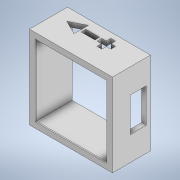
# Autodesk Inventor part: Case
Saved by Autodesk Inventor 2020.1 (Build 241239000, 239)
## iProperties
Created: 2019-09-02
Part Number: Case
Material: Generic
Document SubType Name: Modeling
Designer: matteo.spadetto-1
Density: 1 g/cm^3
Appearance: Default
Author: matteo.spadetto-1
Autodesk Inventor part; units mm, degrees
ref_plane "YZ Plane" through (0, 0, 0) normal (1, 0, 0) x (0, 1, 0)
ref_plane "XZ Plane" through (0, 0, 0) normal (0, 1, 0) x (-1, 0, 0)
ref_plane "XY Plane" through (0, 0, 0) normal (0, 0, 1) x (1, 0, 0)
sketch "Sketch2" plane through (0, 0, 0) normal (0, 0, 1) x (1, 0, 0)
  line L0 (0, 0) -> (73, 0)
  line L1 (73, 0) -> (73, 73)
  line L2 (73, 73) -> (0, 73)
  line L3 (0, 73) -> (0, 0)
  dimension "d2" = 73
  dimension "d3" = 73
  constraints: 8 end point, 2 parallel, 1 horizontal, 1 perpendicular
  measures "d2" distance of L2.end L1.end
  measures "d3" distance of L1.end L0.end
extrude "Extrusion1" add sketch "Sketch2" along normal blind 20
sketch "Sketch3" plane through (0, 0, 0) normal (0, 0, -1) x (-1, 0, 0)
  line L0 (-73, 73) -> (0, 73) projected
  line L1 (0, 73) -> (0, 0) projected
  line L2 (-73, 73) -> (0, 73)
  line L3 (0, 73) -> (0, 0)
  line L4 (0, 0) -> (-73, 0)
  line L5 (-73, 0) -> (-73, 73)
  line L6 (-69, 69) -> (-4, 69)
  line L7 (-4, 69) -> (-4, 4)
  line L8 (-4, 4) -> (-69, 4)
  line L9 (-69, 4) -> (-69, 69)
  dimension "d6" = 4
  constraints: 16 end point, 4 parallel, 2 perpendicular, 1 horizontal, 3 other
  measures "d6" distance between parallel lines of L5 L9
extrude "Extrusion2" cut sketch "Sketch3" against normal blind 20 contours L6 L7 L8 L9
sketch "Sketch4" plane through (0, 0, 20) normal (0, 0, 1) x (1, 0, 0)
  line L0 (4, 4) -> (4, 69) projected
  line L1 (69, 69) -> (69, 4) projected
  line L2 (4, 4) -> (69, 4)
  line L3 (69, 4) -> (69, 69)
  line L4 (69, 69) -> (4, 69)
  line L5 (4, 69) -> (4, 4)
  line L6 (5, 68) -> (68, 68)
  line L7 (68, 68) -> (68, 5)
  line L8 (68, 5) -> (5, 5)
  line L9 (5, 5) -> (5, 68)
  point P0 (0, 0)
  point P1 (69, 4)
  point P2 (4, 69)
  dimension "d9" = 1
  constraints: 16 end point, 4 parallel, 2 perpendicular, 1 horizontal, 3 other
  measures "d9" distance between parallel lines of L4 L6
extrude "Extrusion3" add sketch "Sketch4" against normal blind 1
sketch "Sketch5" plane through (0, 0, 0) normal (0, 0, -1) x (-1, 0, 0)
  line L0 (-4, 69) -> (-4, 4) projected
  line L1 (-4, 4) -> (-69, 4) projected
  line L2 (-4, 69) -> (-69, 69)
  line L3 (-69, 69) -> (-69, 4)
  line L4 (-69, 4) -> (-4, 4)
  line L5 (-4, 4) -> (-4, 69)
  line L6 (0, 73) -> (0, 0) projected
  line L7 (0, 0) -> (-73, 0) projected
  line L8 (0, 73) -> (-73, 73)
  line L9 (-73, 73) -> (-73, 0)
  line L10 (-73, 0) -> (0, 0)
  line L11 (0, 0) -> (0, 73)
  constraints: 16 end point, 4 parallel, 2 horizontal, 2 perpendicular
extrude "Extrusion4" add sketch "Sketch5" along normal blind 13.5
sketch "Sketch7" plane through (73, 0, 20) normal (1, 0, 0) x (0, 0, -1)
  line L0 (33.5, 69) -> (33.5, 4) projected
  line L1 (29.6, 36.5) -> (29.6, 51.5)
  line L2 (29.6, 51.5) -> (15.6, 51.5)
  line L3 (15.6, 51.5) -> (15.6, 21.5)
  line L4 (15.6, 21.5) -> (29.6, 21.5)
  line L5 (29.6, 21.5) -> (29.6, 36.5)
  point P0 (20, 0)
  dimension "d57" = 2.5
  dimension "d43" = 15
  dimension "d44" = 14
  dimension "d45" = 30
  constraints: 10 end point, 3 perpendicular, 1 point on line, 1 vertical
  measures "d43" distance of L1.start L1.end
  measures "d44" distance of L1.end L2.end
  measures "d45" distance of L2.end L3.end
extrude "Extrusion5" cut sketch "Sketch7" against normal blind 4
sketch "Sketch8" plane through (0, 0, 20) normal (-1, 0, 0) x (0, 0, 1)
  line L0 (-26.5, 65) -> (-24, 65)
  circle A0 centre (-24, 65) radius 1.5
  point P0 (-20, 0)
  point P1 (-33.5, 69)
  constraints: 2 end point, 1 centre point, 1 coincident, 1 horizontal
extrude "Extrusion6" cut sketch "Sketch8" against normal blind 4
sketch "Sketch9" plane through (0, 0, 20) normal (-1, 0, 0) x (0, 0, 1)
  line L0 (-33.5, 73) -> (0, 73) projected
  line L1 (-33.5, 73) -> (-33.5, 66.5)
  line L2 (-33.5, 66.5) -> (-31.5, 66.5)
  line L3 (-31.5, 66.5) -> (-31.5, 63.5)
  line L4 (-31.5, 63.5) -> (-33.5, 63.5)
  line L5 (-33.5, 63.5) -> (-33.5, 66.5)
  point P0 (-20, 0)
  dimension "d55" = 2
  dimension "d56" = 3
  constraints: 10 end point, 2 parallel, 1 horizontal, 1 perpendicular, 1 vertical
  measures "d55" distance of L3.end L4.end
  measures "d56" distance of L2.end L3.end
extrude "Extrusion7" cut sketch "Sketch9" against normal blind 2.5
sketch "Sketch10" plane through (0, 73, 20) normal (0, 1, 0) x (1, 0, 0)
  line L0 (0, 0) -> (73, 0) projected
  line L1 (73, 33.5) -> (0, 33.5) projected
  line L2 (0, 33.5) -> (0, 0) projected
  line L3 (4, 33.5) -> (4, 1) projected
  line L4 (51.2, 20.4) -> (47.2, 20.4)
  line L5 (47.2, 20.4) -> (47.2, 16.4)
  line L6 (47.2, 16.4) -> (42.8, 16.4)
  line L7 (42.8, 16.4) -> (42.8, 20.4)
  line L8 (42.8, 20.4) -> (38.8, 20.4)
  line L9 (38.8, 20.4) -> (38.8, 24.8)
  line L10 (38.8, 24.8) -> (42.8, 24.8)
  line L11 (42.8, 24.8) -> (42.8, 28.8)
  line L12 (42.8, 28.8) -> (47.2, 28.8)
  line L13 (47.2, 28.8) -> (47.2, 24.8)
  line L14 (47.2, 24.8) -> (51.2, 24.8)
  line L15 (51.2, 24.8) -> (51.2, 20.4)
  line L16 (24.8, 20.4) -> (37.2, 20.4)
  line L17 (37.2, 20.4) -> (37.2, 24.8)
  line L18 (37.2, 24.8) -> (24.8, 24.8)
  line L19 (24.8, 24.8) -> (24.8, 20.4)
  line L20 (10.161, 22.4041) -> (23.2, 28.9236)
  line L21 (23.2, 28.9236) -> (23.2, 15.8846)
  line L22 (23.2, 15.8846) -> (10.161, 22.4041)
  line L23 (23.1, 28.7618) -> (10.3846, 22.4041)
  line L24 (10.3846, 22.4041) -> (23.1, 16.0464)
  line L25 (23.1, 16.0464) -> (23.1, 28.7618)
  line L26 (24.9, 24.7) -> (37.1, 24.7)
  line L27 (37.1, 24.7) -> (37.1, 20.5)
  line L28 (37.1, 20.5) -> (24.9, 20.5)
  line L29 (24.9, 20.5) -> (24.9, 24.7)
  line L30 (42.9, 24.7) -> (38.9, 24.7)
  line L31 (38.9, 24.7) -> (38.9, 20.5)
  line L32 (38.9, 20.5) -> (42.9, 20.5)
  line L33 (42.9, 20.5) -> (42.9, 16.5)
  line L34 (42.9, 16.5) -> (47.1, 16.5)
  line L35 (47.1, 16.5) -> (47.1, 20.5)
  line L36 (47.1, 20.5) -> (51.1, 20.5)
  line L37 (51.1, 20.5) -> (51.1, 24.7)
  line L38 (51.1, 24.7) -> (47.1, 24.7)
  line L39 (47.1, 24.7) -> (47.1, 28.7)
  line L40 (47.1, 28.7) -> (42.9, 28.7)
  line L41 (42.9, 28.7) -> (42.9, 24.7)
  point P0 (0, 20)
  dimension "d95" = 0.1
  dimension "d96" = 0.1
  dimension "d97" = 0.1
  constraints: 76 end point, 8 perpendicular, 2 parallel, 16 other
  measures "d95" distance between parallel lines of L20 L23
  measures "d96" distance between parallel lines of L18 L26
  measures "d97" distance between parallel lines of L10 L30
extrude "Extrusion8" cut sketch "Sketch10" against normal blind 4 contours L4 L5 L6 L7 L8 L9 L10 L11 L12 L13 L14 L15 | L19 L18 L17 L16 | L20 L21 L22 | L25 L24 L23 | L26 L27 L28 L29 | L41 L40 L39 L38 L37 L36 L35 L34 L33 L32 L31 L30
extrude "Extrusion9" add sketch "Sketch10" against normal blind 4
body "Solid1"
